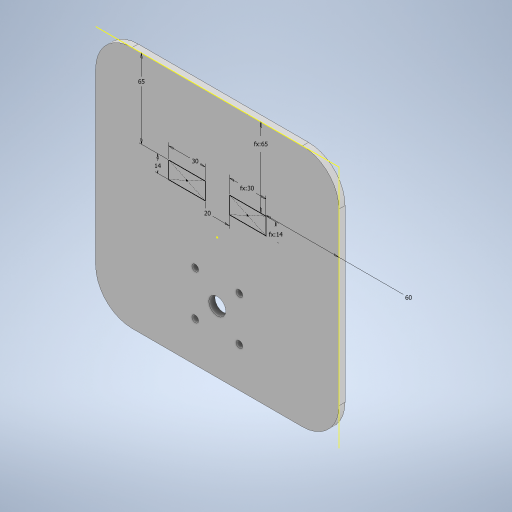
# Autodesk Inventor part: basicmodel
Saved by Autodesk Inventor 2024 (Build 280153000, 153)
## iProperties
Created: 2026-02-19
Part Number: basicmodel
Material: Generic
Document SubType Name: Modeling
Designer: janst
Density: 1 g/cm^3
Appearance: Default
Author: janst
Autodesk Inventor part; units mm, degrees
ref_plane "YZ Plane" through (0, 0, 0) normal (1, 0, 0) x (0, 1, 0)
ref_plane "XZ Plane" through (0, 0, 0) normal (0, 1, 0) x (-1, 0, 0)
ref_plane "XY Plane" through (0, 0, 0) normal (0, 0, 1) x (1, 0, 0)
sketch "Sketch1" plane through (0, 0, 0) normal (0, 0, 1) x (1, 0, 0)
  line L0 (100, -100) -> (-100, -100)
  line L1 (-100, -100) -> (-100, 100)
  line L2 (-100, 100) -> (100, 100)
  line L3 (100, 100) -> (100, -100)
  line L4 (100, -100) -> (-100, 100) construction
  line L5 (-100, -100) -> (100, 100) construction
  point P0 (0, 0)
  dimension "d0" = 200
  dimension "d1" = 200
  constraints: 12 end point, 2 midpoint, 2 parallel, 1 horizontal, 1 perpendicular
  measures "d0" distance of L1.end L2.end
  measures "d1" distance of L2.end L0.start
extrude "Extrusion1" add sketch "Sketch1" along normal blind 5
sketch "Sketch2" plane through (0, 0, 5) normal (0, 0, 1) x (1, 0, 0)
  line L0 (-24.1, -25) -> (24.1, -25)
  line L1 (24.1, -25) -> (24.1, -73.2)
  line L2 (24.1, -73.2) -> (-24.1, -73.2)
  line L3 (-24.1, -73.2) -> (-24.1, -25)
  line L4 (-24.1, -25) -> (24.1, -73.2) construction
  line L5 (24.1, -25) -> (-24.1, -73.2) construction
  line L6 (100, 100) -> (-100, 100) projected
  line L7 (-100, 100) -> (-100, -100) projected
  line L8 (-100, -100) -> (100, -100) projected
  line L9 (100, -100) -> (100, 100) projected
  circle A0 centre (0, -49.1) radius 25.65
  line L10 (24.1, -25) -> (-24.1, -73.2)
  line L11 (-24.1, -25) -> (24.1, -73.2)
  circle A1 centre (0, -49.1) radius 7
  point P0 (0, 0)
  point P1 (-18.1373, -30.9627)
  point P2 (18.1373, -30.9627)
  point P3 (18.1373, -67.2373)
  point P4 (-18.1373, -67.2373)
  dimension "d4" = 48.2
  dimension "d5" = 48.2
  dimension "d6" = 25
  dimension "d7" = 200
  dimension "d8" = 75.9
  dimension "d9" = 51.3
  dimension "d10" = 14
  constraints: 16 end point, 4 point on circle, 4 point on line, 3 equal length, 2 centre point, 2 coincident, 2 midpoint, 1 horizontal, 1 perpendicular
  measures "d4" distance of L0.start L0.end
  measures "d5" distance of L0.end L1.end
  measures "d6" distance from line of point (0, 0) L0
  measures "d7" distance of L7.end L8.end
  measures "d8" distance between parallel lines of L7 L3
  measures "d9" diameter of A0
  measures "d10" diameter of A1
hole "Hole1" at (-18.1373, -30.9627, 5) at (18.1373, -30.9627, 5) at (18.1373, -67.2373, 5) at (-18.1373, -67.2373, 5) direction (0, 0, -1) diameter 5.5 end through all
sketch "Sketch3" plane through (0, 0, 5) normal (0, 0, 1) x (1, 0, 0)
  line L0 (-10, 21) -> (-40, 21)
  line L1 (-40, 21) -> (-40, 35)
  line L2 (-40, 35) -> (-10, 35)
  line L3 (-10, 35) -> (-10, 21)
  line L4 (-10, 21) -> (-40, 35) construction
  line L5 (-40, 21) -> (-10, 35) construction
  line L6 (40, 21) -> (10, 21)
  line L7 (10, 21) -> (10, 35)
  line L8 (10, 35) -> (40, 35)
  line L9 (40, 35) -> (40, 21)
  line L10 (40, 21) -> (10, 35) construction
  line L11 (10, 21) -> (40, 35) construction
  line L12 (100, 100) -> (-100, 100) projected
  line L13 (100, -100) -> (100, 100) projected
  point P0 (0, 0)
  point P1 (-25, 28)
  point P2 (25, 28)
  dimension "d20" = 30
  dimension "d21" = 14
  dimension "d22" = 30
  dimension "d23" = 14
  dimension "d24" = 65
  dimension "d25" = 65
  dimension "d26" = 20
  dimension "d27" = 60
  constraints: 24 end point, 4 midpoint, 4 parallel, 2 horizontal, 2 perpendicular
  measures "d20" distance of L1.end L2.end
  measures "d21" distance of L0.end L1.end
  measures "d22" distance of L7.end L8.end
  measures "d23" distance of L8.end L6.start
  measures "d24" distance between parallel lines of L12 L2
  measures "d25" distance between parallel lines of L12 L8
  measures "d26" distance between parallel lines of L3 L7
  measures "d27" distance between parallel lines of L13 L9
extrude "Extrusion2" cut sketch "Sketch2" against normal blind 5 contours A1 L10 L11 | L11 L10 A1 | L11 A1 L10 | L10 A1 L11
fillet "Fillet1" radius 30 4 edges at (100, 100, 2.5) (100, -100, 2.5) (-100, -100, 2.5) (-100, 100, 2.5)
equation "\"d5\" = d4"
equation "\"d8\" = -0.5 * d4 + 0.5 * d7"
equation "\"d22\" = d20"
equation "\"d23\" = d21"
equation "\"d25\" = d24"
body "Solid1"
